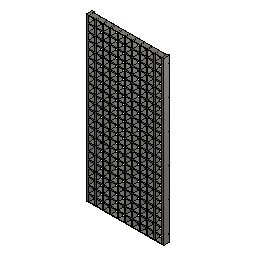
Garlic220 frame (Autodesk Fusion 360 design; units mm, degrees)
Autodesk Fusion 360 part; units mm, degrees
(part 1 of 5)
sketch "Sketch1" plane through (0, 0, 0) normal (0, 0, 1) x (1, 0, 0)
  line L0 (-100, 220) -> (100, 220)
  line L1 (100, 220) -> (100, -220)
  line L2 (100, -220) -> (-100, -220)
  line L3 (-100, -220) -> (-100, 220)
  line L4 (-100, 220) -> (100, -220) construction
  line L5 (100, 220) -> (-100, -220) construction
  line L6 (-100, -220) -> (-80, -220) construction
  line L7 (-80, -220) -> (-80, -200) construction
  line L8 (-80, -200) -> (-100, -200) construction
  line L9 (-100, -200) -> (-100, -220) construction
  line L10 (-98.5, -218.5) -> (-81.5, -218.5)
  line L11 (-81.5, -218.5) -> (-81.5, -201.5)
  line L12 (-81.5, -201.5) -> (-98.5, -201.5)
  line L13 (-98.5, -201.5) -> (-98.5, -218.5)
  line L14 (-61.5, -201.5) -> (-78.5, -201.5)
  line L15 (-61.5, -218.5) -> (-61.5, -201.5)
  line L16 (-78.5, -201.5) -> (-78.5, -218.5)
  line L17 (-78.5, -218.5) -> (-61.5, -218.5)
  line L18 (-60, -220) -> (-60, -200) construction
  line L19 (-60, -200) -> (-80, -200) construction
  line L20 (-41.5, -201.5) -> (-58.5, -201.5)
  line L21 (-41.5, -218.5) -> (-41.5, -201.5)
  line L22 (-58.5, -201.5) -> (-58.5, -218.5)
  line L23 (-58.5, -218.5) -> (-41.5, -218.5)
  line L24 (-40, -220) -> (-40, -200) construction
  line L25 (-40, -200) -> (-60, -200) construction
  line L26 (-21.5, -201.5) -> (-38.5, -201.5)
  line L27 (-21.5, -218.5) -> (-21.5, -201.5)
  line L28 (-38.5, -201.5) -> (-38.5, -218.5)
  line L29 (-38.5, -218.5) -> (-21.5, -218.5)
  line L30 (-20, -220) -> (-20, -200) construction
  line L31 (-20, -200) -> (-40, -200) construction
  line L32 (-1.5, -201.5) -> (-18.5, -201.5)
  line L33 (-1.5, -218.5) -> (-1.5, -201.5)
  line L34 (-18.5, -201.5) -> (-18.5, -218.5)
  line L35 (-18.5, -218.5) -> (-1.5, -218.5)
  line L36 (0, -220) -> (0, -200) construction
  line L37 (0, -200) -> (-20, -200) construction
  line L38 (18.5, -201.5) -> (1.5, -201.5)
  line L39 (18.5, -218.5) -> (18.5, -201.5)
  line L40 (1.5, -201.5) -> (1.5, -218.5)
  line L41 (1.5, -218.5) -> (18.5, -218.5)
  line L42 (20, -220) -> (20, -200) construction
  line L43 (20, -200) -> (0, -200) construction
  line L44 (38.5, -201.5) -> (21.5, -201.5)
  line L45 (38.5, -218.5) -> (38.5, -201.5)
  line L46 (21.5, -201.5) -> (21.5, -218.5)
  line L47 (21.5, -218.5) -> (38.5, -218.5)
  line L48 (40, -220) -> (40, -200) construction
  line L49 (40, -200) -> (20, -200) construction
  line L50 (58.5, -201.5) -> (41.5, -201.5)
  line L51 (58.5, -218.5) -> (58.5, -201.5)
  line L52 (41.5, -201.5) -> (41.5, -218.5)
  line L53 (41.5, -218.5) -> (58.5, -218.5)
  line L54 (60, -220) -> (60, -200) construction
  line L55 (60, -200) -> (40, -200) construction
  line L56 (78.5, -201.5) -> (61.5, -201.5)
  line L57 (78.5, -218.5) -> (78.5, -201.5)
  line L58 (61.5, -201.5) -> (61.5, -218.5)
  line L59 (61.5, -218.5) -> (78.5, -218.5)
  line L60 (80, -220) -> (80, -200) construction
  line L61 (80, -200) -> (60, -200) construction
  line L62 (98.5, -201.5) -> (81.5, -201.5)
  line L63 (98.5, -218.5) -> (98.5, -201.5)
  line L64 (81.5, -201.5) -> (81.5, -218.5)
  line L65 (81.5, -218.5) -> (98.5, -218.5)
  line L66 (100, -220) -> (100, -200) construction
  line L67 (100, -200) -> (80, -200) construction
  line L68 (-81.5, -181.5) -> (-98.5, -181.5)
  line L69 (-81.5, -198.5) -> (-81.5, -181.5)
  line L70 (-98.5, -181.5) -> (-98.5, -198.5)
  line L71 (-98.5, -198.5) -> (-81.5, -198.5)
  line L72 (-80, -200) -> (-80, -180) construction
  line L73 (-80, -180) -> (-100, -180) construction
  line L74 (-61.5, -181.5) -> (-78.5, -181.5)
  line L75 (-61.5, -198.5) -> (-61.5, -181.5)
  line L76 (-78.5, -181.5) -> (-78.5, -198.5)
  line L77 (-78.5, -198.5) -> (-61.5, -198.5)
  line L78 (-60, -200) -> (-60, -180) construction
  line L79 (-60, -180) -> (-80, -180) construction
  line L80 (-41.5, -181.5) -> (-58.5, -181.5)
  line L81 (-41.5, -198.5) -> (-41.5, -181.5)
  line L82 (-58.5, -181.5) -> (-58.5, -198.5)
  line L83 (-58.5, -198.5) -> (-41.5, -198.5)
  line L84 (-40, -200) -> (-40, -180) construction
  line L85 (-40, -180) -> (-60, -180) construction
  line L86 (-21.5, -181.5) -> (-38.5, -181.5)
  line L87 (-21.5, -198.5) -> (-21.5, -181.5)
  line L88 (-38.5, -181.5) -> (-38.5, -198.5)
  line L89 (-38.5, -198.5) -> (-21.5, -198.5)
  line L90 (-20, -200) -> (-20, -180) construction
  line L91 (-20, -180) -> (-40, -180) construction
  line L92 (-1.5, -181.5) -> (-18.5, -181.5)
  line L93 (-1.5, -198.5) -> (-1.5, -181.5)
  line L94 (-18.5, -181.5) -> (-18.5, -198.5)
  line L95 (-18.5, -198.5) -> (-1.5, -198.5)
  line L96 (0, -200) -> (0, -180) construction
  line L97 (0, -180) -> (-20, -180) construction
  line L98 (18.5, -181.5) -> (1.5, -181.5)
  line L99 (18.5, -198.5) -> (18.5, -181.5)
  line L100 (1.5, -181.5) -> (1.5, -198.5)
  line L101 (1.5, -198.5) -> (18.5, -198.5)
  line L102 (20, -200) -> (20, -180) construction
  line L103 (20, -180) -> (0, -180) construction
  line L104 (38.5, -181.5) -> (21.5, -181.5)
  line L105 (38.5, -198.5) -> (38.5, -181.5)
  line L106 (21.5, -181.5) -> (21.5, -198.5)
  line L107 (21.5, -198.5) -> (38.5, -198.5)
  line L108 (40, -200) -> (40, -180) construction
  line L109 (40, -180) -> (20, -180) construction
  line L110 (58.5, -181.5) -> (41.5, -181.5)
  line L111 (58.5, -198.5) -> (58.5, -181.5)
  line L112 (41.5, -181.5) -> (41.5, -198.5)
  line L113 (41.5, -198.5) -> (58.5, -198.5)
  line L114 (60, -200) -> (60, -180) construction
  line L115 (60, -180) -> (40, -180) construction
  line L116 (78.5, -181.5) -> (61.5, -181.5)
  line L117 (78.5, -198.5) -> (78.5, -181.5)
  line L118 (61.5, -181.5) -> (61.5, -198.5)
  line L119 (61.5, -198.5) -> (78.5, -198.5)
  line L120 (80, -200) -> (80, -180) construction
  line L121 (80, -180) -> (60, -180) construction
  line L122 (98.5, -181.5) -> (81.5, -181.5)
  line L123 (98.5, -198.5) -> (98.5, -181.5)
  line L124 (81.5, -181.5) -> (81.5, -198.5)
  line L125 (81.5, -198.5) -> (98.5, -198.5)
  line L126 (100, -200) -> (100, -180) construction
  line L127 (100, -180) -> (80, -180) construction
  line L128 (-81.5, -161.5) -> (-98.5, -161.5)
  line L129 (-81.5, -178.5) -> (-81.5, -161.5)
  line L130 (-98.5, -161.5) -> (-98.5, -178.5)
  line L131 (-98.5, -178.5) -> (-81.5, -178.5)
  line L132 (-80, -180) -> (-80, -160) construction
  line L133 (-80, -160) -> (-100, -160) construction
  line L134 (-61.5, -161.5) -> (-78.5, -161.5)
  line L135 (-61.5, -178.5) -> (-61.5, -161.5)
  line L136 (-78.5, -161.5) -> (-78.5, -178.5)
  line L137 (-78.5, -178.5) -> (-61.5, -178.5)
  line L138 (-60, -180) -> (-60, -160) construction
  line L139 (-60, -160) -> (-80, -160) construction
  line L140 (-41.5, -161.5) -> (-58.5, -161.5)
  line L141 (-41.5, -178.5) -> (-41.5, -161.5)
  line L142 (-58.5, -161.5) -> (-58.5, -178.5)
  line L143 (-58.5, -178.5) -> (-41.5, -178.5)
  line L144 (-40, -180) -> (-40, -160) construction
  line L145 (-40, -160) -> (-60, -160) construction
  line L146 (-21.5, -161.5) -> (-38.5, -161.5)
  line L147 (-21.5, -178.5) -> (-21.5, -161.5)
  line L148 (-38.5, -161.5) -> (-38.5, -178.5)
  line L149 (-38.5, -178.5) -> (-21.5, -178.5)
  line L150 (-20, -180) -> (-20, -160) construction
  line L151 (-20, -160) -> (-40, -160) construction
  line L152 (-1.5, -161.5) -> (-18.5, -161.5)
  line L153 (-1.5, -178.5) -> (-1.5, -161.5)
  line L154 (-18.5, -161.5) -> (-18.5, -178.5)
  line L155 (-18.5, -178.5) -> (-1.5, -178.5)
  line L156 (0, -180) -> (0, -160) construction
  line L157 (0, -160) -> (-20, -160) construction
  line L158 (18.5, -161.5) -> (1.5, -161.5)
  line L159 (18.5, -178.5) -> (18.5, -161.5)
  line L160 (1.5, -161.5) -> (1.5, -178.5)
  line L161 (1.5, -178.5) -> (18.5, -178.5)
  line L162 (20, -180) -> (20, -160) construction
  line L163 (20, -160) -> (0, -160) construction
  line L164 (38.5, -161.5) -> (21.5, -161.5)
  line L165 (38.5, -178.5) -> (38.5, -161.5)
  line L166 (21.5, -161.5) -> (21.5, -178.5)
  line L167 (21.5, -178.5) -> (38.5, -178.5)
  line L168 (40, -180) -> (40, -160) construction
  line L169 (40, -160) -> (20, -160) construction
  line L170 (58.5, -161.5) -> (41.5, -161.5)
  line L171 (58.5, -178.5) -> (58.5, -161.5)
  line L172 (41.5, -161.5) -> (41.5, -178.5)
  line L173 (41.5, -178.5) -> (58.5, -178.5)
  line L174 (60, -180) -> (60, -160) construction
  line L175 (60, -160) -> (40, -160) construction
  line L176 (78.5, -161.5) -> (61.5, -161.5)
  line L177 (78.5, -178.5) -> (78.5, -161.5)
  line L178 (61.5, -161.5) -> (61.5, -178.5)
  line L179 (61.5, -178.5) -> (78.5, -178.5)
  line L180 (80, -180) -> (80, -160) construction
  line L181 (80, -160) -> (60, -160) construction
  line L182 (98.5, -161.5) -> (81.5, -161.5)
  line L183 (98.5, -178.5) -> (98.5, -161.5)
  line L184 (81.5, -161.5) -> (81.5, -178.5)
  line L185 (81.5, -178.5) -> (98.5, -178.5)
  line L186 (100, -180) -> (100, -160) construction
  line L187 (100, -160) -> (80, -160) construction
  line L188 (-81.5, -141.5) -> (-98.5, -141.5)
  line L189 (-81.5, -158.5) -> (-81.5, -141.5)
  line L190 (-98.5, -141.5) -> (-98.5, -158.5)
  line L191 (-98.5, -158.5) -> (-81.5, -158.5)
  line L192 (-80, -160) -> (-80, -140) construction
  line L193 (-80, -140) -> (-100, -140) construction
  line L194 (-61.5, -141.5) -> (-78.5, -141.5)
  line L195 (-61.5, -158.5) -> (-61.5, -141.5)
  line L196 (-78.5, -141.5) -> (-78.5, -158.5)
  line L197 (-78.5, -158.5) -> (-61.5, -158.5)
  line L198 (-60, -160) -> (-60, -140) construction
  line L199 (-60, -140) -> (-80, -140) construction
  line L200 (-41.5, -141.5) -> (-58.5, -141.5)
  line L201 (-41.5, -158.5) -> (-41.5, -141.5)
  line L202 (-58.5, -141.5) -> (-58.5, -158.5)
  line L203 (-58.5, -158.5) -> (-41.5, -158.5)
  line L204 (-40, -160) -> (-40, -140) construction
  line L205 (-40, -140) -> (-60, -140) construction
  line L206 (-21.5, -141.5) -> (-38.5, -141.5)
  line L207 (-21.5, -158.5) -> (-21.5, -141.5)
  line L208 (-38.5, -141.5) -> (-38.5, -158.5)
  line L209 (-38.5, -158.5) -> (-21.5, -158.5)
  line L210 (-20, -160) -> (-20, -140) construction
  line L211 (-20, -140) -> (-40, -140) construction
  line L212 (-1.5, -141.5) -> (-18.5, -141.5)
  line L213 (-1.5, -158.5) -> (-1.5, -141.5)
  line L214 (-18.5, -141.5) -> (-18.5, -158.5)
  line L215 (-18.5, -158.5) -> (-1.5, -158.5)
  line L216 (0, -160) -> (0, -140) construction
  line L217 (0, -140) -> (-20, -140) construction
  line L218 (18.5, -141.5) -> (1.5, -141.5)
  line L219 (18.5, -158.5) -> (18.5, -141.5)
  line L220 (1.5, -141.5) -> (1.5, -158.5)
  line L221 (1.5, -158.5) -> (18.5, -158.5)
  line L222 (20, -160) -> (20, -140) construction
  line L223 (20, -140) -> (0, -140) construction
  line L224 (38.5, -141.5) -> (21.5, -141.5)
  line L225 (38.5, -158.5) -> (38.5, -141.5)
  line L226 (21.5, -141.5) -> (21.5, -158.5)
  line L227 (21.5, -158.5) -> (38.5, -158.5)
  line L228 (40, -160) -> (40, -140) construction
  line L229 (40, -140) -> (20, -140) construction
  line L230 (58.5, -141.5) -> (41.5, -141.5)
  line L231 (58.5, -158.5) -> (58.5, -141.5)
  line L232 (41.5, -141.5) -> (41.5, -158.5)
  line L233 (41.5, -158.5) -> (58.5, -158.5)
  line L234 (60, -160) -> (60, -140) construction
  line L235 (60, -140) -> (40, -140) construction
  line L236 (78.5, -141.5) -> (61.5, -141.5)
  line L237 (78.5, -158.5) -> (78.5, -141.5)
  line L238 (61.5, -141.5) -> (61.5, -158.5)
  line L239 (61.5, -158.5) -> (78.5, -158.5)
  line L240 (80, -160) -> (80, -140) construction
  line L241 (80, -140) -> (60, -140) construction
  line L242 (98.5, -141.5) -> (81.5, -141.5)
  line L243 (98.5, -158.5) -> (98.5, -141.5)
  line L244 (81.5, -141.5) -> (81.5, -158.5)
  line L245 (81.5, -158.5) -> (98.5, -158.5)
  line L246 (100, -160) -> (100, -140) construction
  line L247 (100, -140) -> (80, -140) construction
  line L248 (-81.5, -121.5) -> (-98.5, -121.5)
  line L249 (-81.5, -138.5) -> (-81.5, -121.5)
  line L250 (-98.5, -121.5) -> (-98.5, -138.5)
  line L251 (-98.5, -138.5) -> (-81.5, -138.5)
  line L252 (-80, -140) -> (-80, -120) construction
  line L253 (-80, -120) -> (-100, -120) construction
  line L254 (-61.5, -121.5) -> (-78.5, -121.5)
  line L255 (-61.5, -138.5) -> (-61.5, -121.5)
  line L256 (-78.5, -121.5) -> (-78.5, -138.5)
  line L257 (-78.5, -138.5) -> (-61.5, -138.5)
  line L258 (-60, -140) -> (-60, -120) construction
  line L259 (-60, -120) -> (-80, -120) construction
  line L260 (-41.5, -121.5) -> (-58.5, -121.5)
  line L261 (-41.5, -138.5) -> (-41.5, -121.5)
  line L262 (-58.5, -121.5) -> (-58.5, -138.5)
  line L263 (-58.5, -138.5) -> (-41.5, -138.5)
  line L264 (-40, -140) -> (-40, -120) construction
  line L265 (-40, -120) -> (-60, -120) construction
  line L266 (-21.5, -121.5) -> (-38.5, -121.5)
  line L267 (-21.5, -138.5) -> (-21.5, -121.5)
  line L268 (-38.5, -121.5) -> (-38.5, -138.5)
  line L269 (-38.5, -138.5) -> (-21.5, -138.5)
  line L270 (-20, -140) -> (-20, -120) construction
  line L271 (-20, -120) -> (-40, -120) construction
  line L272 (-1.5, -121.5) -> (-18.5, -121.5)
  line L273 (-1.5, -138.5) -> (-1.5, -121.5)
  line L274 (-18.5, -121.5) -> (-18.5, -138.5)
  line L275 (-18.5, -138.5) -> (-1.5, -138.5)
  line L276 (0, -140) -> (0, -120) construction
  line L277 (0, -120) -> (-20, -120) construction
  line L278 (18.5, -121.5) -> (1.5, -121.5)
  line L279 (18.5, -138.5) -> (18.5, -121.5)
  line L280 (1.5, -121.5) -> (1.5, -138.5)
  line L281 (1.5, -138.5) -> (18.5, -138.5)
  line L282 (20, -140) -> (20, -120) construction
  line L283 (20, -120) -> (0, -120) construction
  line L284 (38.5, -121.5) -> (21.5, -121.5)
  line L285 (38.5, -138.5) -> (38.5, -121.5)
  line L286 (21.5, -121.5) -> (21.5, -138.5)
  line L287 (21.5, -138.5) -> (38.5, -138.5)
  line L288 (40, -140) -> (40, -120) construction
  line L289 (40, -120) -> (20, -120) construction
  line L290 (58.5, -121.5) -> (41.5, -121.5)
  line L291 (58.5, -138.5) -> (58.5, -121.5)
  line L292 (41.5, -121.5) -> (41.5, -138.5)
  line L293 (41.5, -138.5) -> (58.5, -138.5)
  line L294 (60, -140) -> (60, -120) construction
  line L295 (60, -120) -> (40, -120) construction
  line L296 (78.5, -121.5) -> (61.5, -121.5)
  line L297 (78.5, -138.5) -> (78.5, -121.5)
  line L298 (61.5, -121.5) -> (61.5, -138.5)
  line L299 (61.5, -138.5) -> (78.5, -138.5)
  line L300 (80, -140) -> (80, -120) construction
  line L301 (80, -120) -> (60, -120) construction
  line L302 (98.5, -121.5) -> (81.5, -121.5)
  line L303 (98.5, -138.5) -> (98.5, -121.5)
  line L304 (81.5, -121.5) -> (81.5, -138.5)
  line L305 (81.5, -138.5) -> (98.5, -138.5)
  line L306 (100, -140) -> (100, -120) construction
  line L307 (100, -120) -> (80, -120) construction
  line L308 (-81.5, -101.5) -> (-98.5, -101.5)
  line L309 (-81.5, -118.5) -> (-81.5, -101.5)
  line L310 (-98.5, -101.5) -> (-98.5, -118.5)
  line L311 (-98.5, -118.5) -> (-81.5, -118.5)
  line L312 (-80, -120) -> (-80, -100) construction
  line L313 (-80, -100) -> (-100, -100) construction
  line L314 (-61.5, -101.5) -> (-78.5, -101.5)
  line L315 (-61.5, -118.5) -> (-61.5, -101.5)
  line L316 (-78.5, -101.5) -> (-78.5, -118.5)
  line L317 (-78.5, -118.5) -> (-61.5, -118.5)
  line L318 (-60, -120) -> (-60, -100) construction
  line L319 (-60, -100) -> (-80, -100) construction
  line L320 (-41.5, -101.5) -> (-58.5, -101.5)
  line L321 (-41.5, -118.5) -> (-41.5, -101.5)
  line L322 (-58.5, -101.5) -> (-58.5, -118.5)
  line L323 (-58.5, -118.5) -> (-41.5, -118.5)
  line L324 (-40, -120) -> (-40, -100) construction
  line L325 (-40, -100) -> (-60, -100) construction
  line L326 (-21.5, -101.5) -> (-38.5, -101.5)
  line L327 (-21.5, -118.5) -> (-21.5, -101.5)
  line L328 (-38.5, -101.5) -> (-38.5, -118.5)
  line L329 (-38.5, -118.5) -> (-21.5, -118.5)
  line L330 (-20, -120) -> (-20, -100) construction
  line L331 (-20, -100) -> (-40, -100) construction
  line L332 (-1.5, -101.5) -> (-18.5, -101.5)
  line L333 (-1.5, -118.5) -> (-1.5, -101.5)
  line L334 (-18.5, -101.5) -> (-18.5, -118.5)
  line L335 (-18.5, -118.5) -> (-1.5, -118.5)
  line L336 (0, -120) -> (0, -100) construction
  line L337 (0, -100) -> (-20, -100) construction
  line L338 (18.5, -101.5) -> (1.5, -101.5)
  line L339 (18.5, -118.5) -> (18.5, -101.5)
  line L340 (1.5, -101.5) -> (1.5, -118.5)
  line L341 (1.5, -118.5) -> (18.5, -118.5)
  line L342 (20, -120) -> (20, -100) construction
  line L343 (20, -100) -> (0, -100) construction
  line L344 (38.5, -101.5) -> (21.5, -101.5)
  line L345 (38.5, -118.5) -> (38.5, -101.5)
  line L346 (21.5, -101.5) -> (21.5, -118.5)
  line L347 (21.5, -118.5) -> (38.5, -118.5)
  line L348 (40, -120) -> (40, -100) construction
  line L349 (40, -100) -> (20, -100) construction
  line L350 (58.5, -101.5) -> (41.5, -101.5)
  line L351 (58.5, -118.5) -> (58.5, -101.5)
  line L352 (41.5, -101.5) -> (41.5, -118.5)
  line L353 (41.5, -118.5) -> (58.5, -118.5)
  line L354 (60, -120) -> (60, -100) construction
  line L355 (60, -100) -> (40, -100) construction
  line L356 (78.5, -101.5) -> (61.5, -101.5)
  line L357 (78.5, -118.5) -> (78.5, -101.5)
  line L358 (61.5, -101.5) -> (61.5, -118.5)
  line L359 (61.5, -118.5) -> (78.5, -118.5)
  line L360 (80, -120) -> (80, -100) construction
  line L361 (80, -100) -> (60, -100) construction
  line L362 (98.5, -101.5) -> (81.5, -101.5)
  line L363 (98.5, -118.5) -> (98.5, -101.5)
  line L364 (81.5, -101.5) -> (81.5, -118.5)
  line L365 (81.5, -118.5) -> (98.5, -118.5)
  line L366 (100, -120) -> (100, -100) construction
  line L367 (100, -100) -> (80, -100) construction
  line L368 (-81.5, -81.5) -> (-98.5, -81.5)
  line L369 (-81.5, -98.5) -> (-81.5, -81.5)
  line L370 (-98.5, -81.5) -> (-98.5, -98.5)
  line L371 (-98.5, -98.5) -> (-81.5, -98.5)
  line L372 (-80, -100) -> (-80, -80) construction
  line L373 (-80, -80) -> (-100, -80) construction
  line L374 (-61.5, -81.5) -> (-78.5, -81.5)
  line L375 (-61.5, -98.5) -> (-61.5, -81.5)
  line L376 (-78.5, -81.5) -> (-78.5, -98.5)
  line L377 (-78.5, -98.5) -> (-61.5, -98.5)
  line L378 (-60, -100) -> (-60, -80) construction
  line L379 (-60, -80) -> (-80, -80) construction
  line L380 (-41.5, -81.5) -> (-58.5, -81.5)
  line L381 (-41.5, -98.5) -> (-41.5, -81.5)
  line L382 (-58.5, -81.5) -> (-58.5, -98.5)
  line L383 (-58.5, -98.5) -> (-41.5, -98.5)
  line L384 (-40, -100) -> (-40, -80) construction
  line L385 (-40, -80) -> (-60, -80) construction
  line L386 (-21.5, -81.5) -> (-38.5, -81.5)
  line L387 (-21.5, -98.5) -> (-21.5, -81.5)
  line L388 (-38.5, -81.5) -> (-38.5, -98.5)
  line L389 (-38.5, -98.5) -> (-21.5, -98.5)
  line L390 (-20, -100) -> (-20, -80) construction
  line L391 (-20, -80) -> (-40, -80) construction
  line L392 (-1.5, -81.5) -> (-18.5, -81.5)
  line L393 (-1.5, -98.5) -> (-1.5, -81.5)
  line L394 (-18.5, -81.5) -> (-18.5, -98.5)
  line L395 (-18.5, -98.5) -> (-1.5, -98.5)
  line L396 (0, -100) -> (0, -80) construction
  line L397 (0, -80) -> (-20, -80) construction
  line L398 (18.5, -81.5) -> (1.5, -81.5)
  line L399 (18.5, -98.5) -> (18.5, -81.5)
  line L400 (1.5, -81.5) -> (1.5, -98.5)
  line L401 (1.5, -98.5) -> (18.5, -98.5)
  line L402 (20, -100) -> (20, -80) construction
  line L403 (20, -80) -> (0, -80) construction
  line L404 (38.5, -81.5) -> (21.5, -81.5)
  line L405 (38.5, -98.5) -> (38.5, -81.5)
  line L406 (21.5, -81.5) -> (21.5, -98.5)
  line L407 (21.5, -98.5) -> (38.5, -98.5)
  line L408 (40, -100) -> (40, -80) construction
  line L409 (40, -80) -> (20, -80) construction
  line L410 (58.5, -81.5) -> (41.5, -81.5)
  line L411 (58.5, -98.5) -> (58.5, -81.5)
  line L412 (41.5, -81.5) -> (41.5, -98.5)
  line L413 (41.5, -98.5) -> (58.5, -98.5)
  line L414 (60, -100) -> (60, -80) construction
  line L415 (60, -80) -> (40, -80) construction
  line L416 (78.5, -81.5) -> (61.5, -81.5)
  line L417 (78.5, -98.5) -> (78.5, -81.5)
  line L418 (61.5, -81.5) -> (61.5, -98.5)
  line L419 (61.5, -98.5) -> (78.5, -98.5)
  line L420 (80, -100) -> (80, -80) construction
  line L421 (80, -80) -> (60, -80) construction
  line L422 (98.5, -81.5) -> (81.5, -81.5)
  line L423 (98.5, -98.5) -> (98.5, -81.5)
  line L424 (81.5, -81.5) -> (81.5, -98.5)
  line L425 (81.5, -98.5) -> (98.5, -98.5)
  line L426 (100, -100) -> (100, -80) construction
  line L427 (100, -80) -> (80, -80) construction
  line L428 (-81.5, -61.5) -> (-98.5, -61.5)
  line L429 (-81.5, -78.5) -> (-81.5, -61.5)
  line L430 (-98.5, -61.5) -> (-98.5, -78.5)
  line L431 (-98.5, -78.5) -> (-81.5, -78.5)
  line L432 (-80, -80) -> (-80, -60) construction
  line L433 (-80, -60) -> (-100, -60) construction
  line L434 (-61.5, -61.5) -> (-78.5, -61.5)
  line L435 (-61.5, -78.5) -> (-61.5, -61.5)
  line L436 (-78.5, -61.5) -> (-78.5, -78.5)
  line L437 (-78.5, -78.5) -> (-61.5, -78.5)
  line L438 (-60, -80) -> (-60, -60) construction
  line L439 (-60, -60) -> (-80, -60) construction
  line L440 (-41.5, -61.5) -> (-58.5, -61.5)
  line L441 (-41.5, -78.5) -> (-41.5, -61.5)
  line L442 (-58.5, -61.5) -> (-58.5, -78.5)
  line L443 (-58.5, -78.5) -> (-41.5, -78.5)
  line L444 (-40, -80) -> (-40, -60) construction
  line L445 (-40, -60) -> (-60, -60) construction
  line L446 (-21.5, -61.5) -> (-38.5, -61.5)
  line L447 (-21.5, -78.5) -> (-21.5, -61.5)
  line L448 (-38.5, -61.5) -> (-38.5, -78.5)
  line L449 (-38.5, -78.5) -> (-21.5, -78.5)
  line L450 (-20, -80) -> (-20, -60) construction
  line L451 (-20, -60) -> (-40, -60) construction
  line L452 (-1.5, -61.5) -> (-18.5, -61.5)
  line L453 (-1.5, -78.5) -> (-1.5, -61.5)
  line L454 (-18.5, -61.5) -> (-18.5, -78.5)
  line L455 (-18.5, -78.5) -> (-1.5, -78.5)
  line L456 (0, -80) -> (0, -60) construction
  line L457 (0, -60) -> (-20, -60) construction
  line L458 (18.5, -61.5) -> (1.5, -61.5)
  line L459 (18.5, -78.5) -> (18.5, -61.5)
  line L460 (1.5, -61.5) -> (1.5, -78.5)
  line L461 (1.5, -78.5) -> (18.5, -78.5)
  line L462 (20, -80) -> (20, -60) construction
  line L463 (20, -60) -> (0, -60) construction
  line L464 (38.5, -61.5) -> (21.5, -61.5)
  line L465 (38.5, -78.5) -> (38.5, -61.5)
  line L466 (21.5, -61.5) -> (21.5, -78.5)
  line L467 (21.5, -78.5) -> (38.5, -78.5)
  line L468 (40, -80) -> (40, -60) construction
  line L469 (40, -60) -> (20, -60) construction
  line L470 (58.5, -61.5) -> (41.5, -61.5)
  line L471 (58.5, -78.5) -> (58.5, -61.5)
  line L472 (41.5, -61.5) -> (41.5, -78.5)
  line L473 (41.5, -78.5) -> (58.5, -78.5)
  line L474 (60, -80) -> (60, -60) construction
  line L475 (60, -60) -> (40, -60) construction
  line L476 (78.5, -61.5) -> (61.5, -61.5)
  line L477 (78.5, -78.5) -> (78.5, -61.5)
  line L478 (61.5, -61.5) -> (61.5, -78.5)
  line L479 (61.5, -78.5) -> (78.5, -78.5)
  line L480 (80, -80) -> (80, -60) construction
  line L481 (80, -60) -> (60, -60) construction
  line L482 (98.5, -61.5) -> (81.5, -61.5)
  line L483 (98.5, -78.5) -> (98.5, -61.5)
  line L484 (81.5, -61.5) -> (81.5, -78.5)
  line L485 (81.5, -78.5) -> (98.5, -78.5)
  line L486 (100, -80) -> (100, -60) construction
  line L487 (100, -60) -> (80, -60) construction
  line L488 (-81.5, -41.5) -> (-98.5, -41.5)
  line L489 (-81.5, -58.5) -> (-81.5, -41.5)
  line L490 (-98.5, -41.5) -> (-98.5, -58.5)
  line L491 (-98.5, -58.5) -> (-81.5, -58.5)
  line L492 (-80, -60) -> (-80, -40) construction
  line L493 (-80, -40) -> (-100, -40) construction
  line L494 (-61.5, -41.5) -> (-78.5, -41.5)
  line L495 (-61.5, -58.5) -> (-61.5, -41.5)
  line L496 (-78.5, -41.5) -> (-78.5, -58.5)
  line L497 (-78.5, -58.5) -> (-61.5, -58.5)
  line L498 (-60, -60) -> (-60, -40) construction
  line L499 (-60, -40) -> (-80, -40) construction
  line L500 (-41.5, -41.5) -> (-58.5, -41.5)
  line L501 (-41.5, -58.5) -> (-41.5, -41.5)
  line L502 (-58.5, -41.5) -> (-58.5, -58.5)
  line L503 (-58.5, -58.5) -> (-41.5, -58.5)
  line L504 (-40, -60) -> (-40, -40) construction
  line L505 (-40, -40) -> (-60, -40) construction
  line L506 (-21.5, -41.5) -> (-38.5, -41.5)
  line L507 (-21.5, -58.5) -> (-21.5, -41.5)
  line L508 (-38.5, -41.5) -> (-38.5, -58.5)
  line L509 (-38.5, -58.5) -> (-21.5, -58.5)
  line L510 (-20, -60) -> (-20, -40) construction
  line L511 (-20, -40) -> (-40, -40) construction
  line L512 (-1.5, -41.5) -> (-18.5, -41.5)
  line L513 (-1.5, -58.5) -> (-1.5, -41.5)
  line L514 (-18.5, -41.5) -> (-18.5, -58.5)
  line L515 (-18.5, -58.5) -> (-1.5, -58.5)
  line L516 (0, -60) -> (0, -40) construction
  line L517 (0, -40) -> (-20, -40) construction
  line L518 (18.5, -41.5) -> (1.5, -41.5)
  line L519 (18.5, -58.5) -> (18.5, -41.5)
  line L520 (1.5, -41.5) -> (1.5, -58.5)
  line L521 (1.5, -58.5) -> (18.5, -58.5)
  line L522 (20, -60) -> (20, -40) construction
  line L523 (20, -40) -> (0, -40) construction
  line L524 (38.5, -41.5) -> (21.5, -41.5)
  line L525 (38.5, -58.5) -> (38.5, -41.5)
  line L526 (21.5, -41.5) -> (21.5, -58.5)
  line L527 (21.5, -58.5) -> (38.5, -58.5)
  line L528 (40, -60) -> (40, -40) construction
  line L529 (40, -40) -> (20, -40) construction
  line L530 (58.5, -41.5) -> (41.5, -41.5)
  line L531 (58.5, -58.5) -> (58.5, -41.5)
  line L532 (41.5, -41.5) -> (41.5, -58.5)
  line L533 (41.5, -58.5) -> (58.5, -58.5)
  line L534 (60, -60) -> (60, -40) construction
  line L535 (60, -40) -> (40, -40) construction
  line L536 (78.5, -41.5) -> (61.5, -41.5)
  line L537 (78.5, -58.5) -> (78.5, -41.5)
  line L538 (61.5, -41.5) -> (61.5, -58.5)
  line L539 (61.5, -58.5) -> (78.5, -58.5)
  line L540 (80, -60) -> (80, -40) construction
  line L541 (80, -40) -> (60, -40) construction
  line L542 (98.5, -41.5) -> (81.5, -41.5)
  line L543 (98.5, -58.5) -> (98.5, -41.5)
  line L544 (81.5, -41.5) -> (81.5, -58.5)
  line L545 (81.5, -58.5) -> (98.5, -58.5)
  line L546 (100, -60) -> (100, -40) construction
  line L547 (100, -40) -> (80, -40) construction
  line L548 (-81.5, -21.5) -> (-98.5, -21.5)
  line L549 (-81.5, -38.5) -> (-81.5, -21.5)
  line L550 (-98.5, -21.5) -> (-98.5, -38.5)
  line L551 (-98.5, -38.5) -> (-81.5, -38.5)
  line L552 (-80, -40) -> (-80, -20) construction
  line L553 (-80, -20) -> (-100, -20) construction
  line L554 (-61.5, -21.5) -> (-78.5, -21.5)
  line L555 (-61.5, -38.5) -> (-61.5, -21.5)
  line L556 (-78.5, -21.5) -> (-78.5, -38.5)
  line L557 (-78.5, -38.5) -> (-61.5, -38.5)
  line L558 (-60, -40) -> (-60, -20) construction
  line L559 (-60, -20) -> (-80, -20) construction
  line L560 (-41.5, -21.5) -> (-58.5, -21.5)
  line L561 (-41.5, -38.5) -> (-41.5, -21.5)
  line L562 (-58.5, -21.5) -> (-58.5, -38.5)
  line L563 (-58.5, -38.5) -> (-41.5, -38.5)
  line L564 (-40, -40) -> (-40, -20) construction
  line L565 (-40, -20) -> (-60, -20) construction
  line L566 (-21.5, -21.5) -> (-38.5, -21.5)
  line L567 (-21.5, -38.5) -> (-21.5, -21.5)
  line L568 (-38.5, -21.5) -> (-38.5, -38.5)
  line L569 (-38.5, -38.5) -> (-21.5, -38.5)
  line L570 (-20, -40) -> (-20, -20) construction
  line L571 (-20, -20) -> (-40, -20) construction
  line L572 (-1.5, -21.5) -> (-18.5, -21.5)
  line L573 (-1.5, -38.5) -> (-1.5, -21.5)
  line L574 (-18.5, -21.5) -> (-18.5, -38.5)
  line L575 (-18.5, -38.5) -> (-1.5, -38.5)
  line L576 (0, -40) -> (0, -20) construction
  line L577 (0, -20) -> (-20, -20) construction
  line L578 (18.5, -21.5) -> (1.5, -21.5)
  line L579 (18.5, -38.5) -> (18.5, -21.5)
  line L580 (1.5, -21.5) -> (1.5, -38.5)
  line L581 (1.5, -38.5) -> (18.5, -38.5)
  line L582 (20, -40) -> (20, -20) construction
  line L583 (20, -20) -> (0, -20) construction
  line L584 (38.5, -21.5) -> (21.5, -21.5)
  line L585 (38.5, -38.5) -> (38.5, -21.5)
  line L586 (21.5, -21.5) -> (21.5, -38.5)
  line L587 (21.5, -38.5) -> (38.5, -38.5)
  line L588 (40, -40) -> (40, -20) construction
  line L589 (40, -20) -> (20, -20) construction
  line L590 (58.5, -21.5) -> (41.5, -21.5)
  line L591 (58.5, -38.5) -> (58.5, -21.5)
  line L592 (41.5, -21.5) -> (41.5, -38.5)
  line L593 (41.5, -38.5) -> (58.5, -38.5)
  line L594 (60, -40) -> (60, -20) construction
  line L595 (60, -20) -> (40, -20) construction
  line L596 (78.5, -21.5) -> (61.5, -21.5)
  line L597 (78.5, -38.5) -> (78.5, -21.5)
  line L598 (61.5, -21.5) -> (61.5, -38.5)
  line L599 (61.5, -38.5) -> (78.5, -38.5)
  line L600 (80, -40) -> (80, -20) construction
  line L601 (80, -20) -> (60, -20) construction
  line L602 (98.5, -21.5) -> (81.5, -21.5)
  line L603 (98.5, -38.5) -> (98.5, -21.5)
  line L604 (81.5, -21.5) -> (81.5, -38.5)
  line L605 (81.5, -38.5) -> (98.5, -38.5)
  line L606 (100, -40) -> (100, -20) construction
  line L607 (100, -20) -> (80, -20) construction
  line L608 (-81.5, -1.5) -> (-98.5, -1.5)
  line L609 (-81.5, -18.5) -> (-81.5, -1.5)
  line L610 (-98.5, -1.5) -> (-98.5, -18.5)
  line L611 (-98.5, -18.5) -> (-81.5, -18.5)
  line L612 (-80, -20) -> (-80, 0) construction
  line L613 (-80, 0) -> (-100, 0) construction
  line L614 (-61.5, -1.5) -> (-78.5, -1.5)
  line L615 (-61.5, -18.5) -> (-61.5, -1.5)
  line L616 (-78.5, -1.5) -> (-78.5, -18.5)
  line L617 (-78.5, -18.5) -> (-61.5, -18.5)
  line L618 (-60, -20) -> (-60, 0) construction
  line L619 (-60, 0) -> (-80, 0) construction
  line L620 (-41.5, -1.5) -> (-58.5, -1.5)
  line L621 (-41.5, -18.5) -> (-41.5, -1.5)
  line L622 (-58.5, -1.5) -> (-58.5, -18.5)
  line L623 (-58.5, -18.5) -> (-41.5, -18.5)
  line L624 (-40, -20) -> (-40, 0) construction
  line L625 (-40, 0) -> (-60, 0) construction
  line L626 (-21.5, -1.5) -> (-38.5, -1.5)
  line L627 (-21.5, -18.5) -> (-21.5, -1.5)
  line L628 (-38.5, -1.5) -> (-38.5, -18.5)
  line L629 (-38.5, -18.5) -> (-21.5, -18.5)
  line L630 (-20, -20) -> (-20, 0) construction
  line L631 (-20, 0) -> (-40, 0) construction
  line L632 (-1.5, -1.5) -> (-18.5, -1.5)
  line L633 (-1.5, -18.5) -> (-1.5, -1.5)
  line L634 (-18.5, -1.5) -> (-18.5, -18.5)
  line L635 (-18.5, -18.5) -> (-1.5, -18.5)
  line L636 (0, -20) -> (0, 0) construction
  line L637 (0, 0) -> (-20, 0) construction
  line L638 (18.5, -1.5) -> (1.5, -1.5)
  line L639 (18.5, -18.5) -> (18.5, -1.5)
  line L640 (1.5, -1.5) -> (1.5, -18.5)
  line L641 (1.5, -18.5) -> (18.5, -18.5)
  line L642 (20, -20) -> (20, 0) construction
  line L643 (20, 0) -> (0, 0) construction
  line L644 (38.5, -1.5) -> (21.5, -1.5)
  line L645 (38.5, -18.5) -> (38.5, -1.5)
  line L646 (21.5, -1.5) -> (21.5, -18.5)
  line L647 (21.5, -18.5) -> (38.5, -18.5)
  line L648 (40, -20) -> (40, 0) construction
  line L649 (40, 0) -> (20, 0) construction
  line L650 (58.5, -1.5) -> (41.5, -1.5)
  line L651 (58.5, -18.5) -> (58.5, -1.5)
  line L652 (41.5, -1.5) -> (41.5, -18.5)
  line L653 (41.5, -18.5) -> (58.5, -18.5)
  line L654 (60, -20) -> (60, 0) construction
  line L655 (60, 0) -> (40, 0) construction
  line L656 (78.5, -1.5) -> (61.5, -1.5)
  line L657 (78.5, -18.5) -> (78.5, -1.5)
  line L658 (61.5, -1.5) -> (61.5, -18.5)
  line L659 (61.5, -18.5) -> (78.5, -18.5)
  line L660 (80, -20) -> (80, 0) construction
  line L661 (80, 0) -> (60, 0) construction
  line L662 (98.5, -1.5) -> (81.5, -1.5)
  line L663 (98.5, -18.5) -> (98.5, -1.5)
  line L664 (81.5, -1.5) -> (81.5, -18.5)
  line L665 (81.5, -18.5) -> (98.5, -18.5)
  line L666 (100, -20) -> (100, 0) construction
  line L667 (100, 0) -> (80, 0) construction
  line L668 (-81.5, 18.5) -> (-98.5, 18.5)
  line L669 (-81.5, 1.5) -> (-81.5, 18.5)
  line L670 (-98.5, 18.5) -> (-98.5, 1.5)
  line L671 (-98.5, 1.5) -> (-81.5, 1.5)
  line L672 (-80, 0) -> (-80, 20) construction
  line L673 (-80, 20) -> (-100, 20) construction
  line L674 (-61.5, 18.5) -> (-78.5, 18.5)
  line L675 (-61.5, 1.5) -> (-61.5, 18.5)
  line L676 (-78.5, 18.5) -> (-78.5, 1.5)
  line L677 (-78.5, 1.5) -> (-61.5, 1.5)
  line L678 (-60, 0) -> (-60, 20) construction
  line L679 (-60, 20) -> (-80, 20) construction
  line L680 (-41.5, 18.5) -> (-58.5, 18.5)
  line L681 (-41.5, 1.5) -> (-41.5, 18.5)
  line L682 (-58.5, 18.5) -> (-58.5, 1.5)
  line L683 (-58.5, 1.5) -> (-41.5, 1.5)
  line L684 (-40, 0) -> (-40, 20) construction
  line L685 (-40, 20) -> (-60, 20) construction
  line L686 (-21.5, 18.5) -> (-38.5, 18.5)
  line L687 (-21.5, 1.5) -> (-21.5, 18.5)
  line L688 (-38.5, 18.5) -> (-38.5, 1.5)
  line L689 (-38.5, 1.5) -> (-21.5, 1.5)
  line L690 (-20, 0) -> (-20, 20) construction
  line L691 (-20, 20) -> (-40, 20) construction
  line L692 (-1.5, 18.5) -> (-18.5, 18.5)
  line L693 (-1.5, 1.5) -> (-1.5, 18.5)
  line L694 (-18.5, 18.5) -> (-18.5, 1.5)
  line L695 (-18.5, 1.5) -> (-1.5, 1.5)
  line L696 (0, 0) -> (0, 20) construction
  line L697 (0, 20) -> (-20, 20) construction
  line L698 (18.5, 18.5) -> (1.5, 18.5)
  line L699 (18.5, 1.5) -> (18.5, 18.5)
  line L700 (1.5, 18.5) -> (1.5, 1.5)
  line L701 (1.5, 1.5) -> (18.5, 1.5)
  line L702 (20, 0) -> (20, 20) construction
  line L703 (20, 20) -> (0, 20) construction
  line L704 (38.5, 18.5) -> (21.5, 18.5)
  line L705 (38.5, 1.5) -> (38.5, 18.5)
  line L706 (21.5, 18.5) -> (21.5, 1.5)
  line L707 (21.5, 1.5) -> (38.5, 1.5)
  line L708 (40, 0) -> (40, 20) construction
  line L709 (40, 20) -> (20, 20) construction
  line L710 (58.5, 18.5) -> (41.5, 18.5)
  line L711 (58.5, 1.5) -> (58.5, 18.5)
  line L712 (41.5, 18.5) -> (41.5, 1.5)
  line L713 (41.5, 1.5) -> (58.5, 1.5)
  line L714 (60, 0) -> (60, 20) construction
  line L715 (60, 20) -> (40, 20) construction
  line L716 (78.5, 18.5) -> (61.5, 18.5)
  line L717 (78.5, 1.5) -> (78.5, 18.5)
  line L718 (61.5, 18.5) -> (61.5, 1.5)
  line L719 (61.5, 1.5) -> (78.5, 1.5)
  line L720 (80, 0) -> (80, 20) construction
  line L721 (80, 20) -> (60, 20) construction
  line L722 (98.5, 18.5) -> (81.5, 18.5)
  line L723 (98.5, 1.5) -> (98.5, 18.5)
  line L724 (81.5, 18.5) -> (81.5, 1.5)
  line L725 (81.5, 1.5) -> (98.5, 1.5)
  line L726 (100, 0) -> (100, 20) construction
  line L727 (100, 20) -> (80, 20) construction
  line L728 (-81.5, 38.5) -> (-98.5, 38.5)
  line L729 (-81.5, 21.5) -> (-81.5, 38.5)
  line L730 (-98.5, 38.5) -> (-98.5, 21.5)
  line L731 (-98.5, 21.5) -> (-81.5, 21.5)
  line L732 (-80, 20) -> (-80, 40) construction
  line L733 (-80, 40) -> (-100, 40) construction
  line L734 (-61.5, 38.5) -> (-78.5, 38.5)
  line L735 (-61.5, 21.5) -> (-61.5, 38.5)
  line L736 (-78.5, 38.5) -> (-78.5, 21.5)
  line L737 (-78.5, 21.5) -> (-61.5, 21.5)
  line L738 (-60, 20) -> (-60, 40) construction
  line L739 (-60, 40) -> (-80, 40) construction
  line L740 (-41.5, 38.5) -> (-58.5, 38.5)
  line L741 (-41.5, 21.5) -> (-41.5, 38.5)
  line L742 (-58.5, 38.5) -> (-58.5, 21.5)
  line L743 (-58.5, 21.5) -> (-41.5, 21.5)
  line L744 (-40, 20) -> (-40, 40) construction
  line L745 (-40, 40) -> (-60, 40) construction
  line L746 (-21.5, 38.5) -> (-38.5, 38.5)
  line L747 (-21.5, 21.5) -> (-21.5, 38.5)
  line L748 (-38.5, 38.5) -> (-38.5, 21.5)
  line L749 (-38.5, 21.5) -> (-21.5, 21.5)
  line L750 (-20, 20) -> (-20, 40) construction
  line L751 (-20, 40) -> (-40, 40) construction
  line L752 (-1.5, 38.5) -> (-18.5, 38.5)
  line L753 (-1.5, 21.5) -> (-1.5, 38.5)
  line L754 (-18.5, 38.5) -> (-18.5, 21.5)
  line L755 (-18.5, 21.5) -> (-1.5, 21.5)
  line L756 (0, 20) -> (0, 40) construction
  line L757 (0, 40) -> (-20, 40) construction
  line L758 (18.5, 38.5) -> (1.5, 38.5)
  line L759 (18.5, 21.5) -> (18.5, 38.5)
  line L760 (1.5, 38.5) -> (1.5, 21.5)
  line L761 (1.5, 21.5) -> (18.5, 21.5)
  line L762 (20, 20) -> (20, 40) construction
  line L763 (20, 40) -> (0, 40) construction
  line L764 (38.5, 38.5) -> (21.5, 38.5)
  line L765 (38.5, 21.5) -> (38.5, 38.5)
  line L766 (21.5, 38.5) -> (21.5, 21.5)
  line L767 (21.5, 21.5) -> (38.5, 21.5)
  line L768 (40, 20) -> (40, 40) construction
  line L769 (40, 40) -> (20, 40) construction
  line L770 (58.5, 38.5) -> (41.5, 38.5)
  line L771 (58.5, 21.5) -> (58.5, 38.5)
  line L772 (41.5, 38.5) -> (41.5, 21.5)
  line L773 (41.5, 21.5) -> (58.5, 21.5)
  line L774 (60, 20) -> (60, 40) construction
  line L775 (60, 40) -> (40, 40) construction
  line L776 (78.5, 38.5) -> (61.5, 38.5)
  line L777 (78.5, 21.5) -> (78.5, 38.5)
  line L778 (61.5, 38.5) -> (61.5, 21.5)
  line L779 (61.5, 21.5) -> (78.5, 21.5)
  line L780 (80, 20) -> (80, 40) construction
  line L781 (80, 40) -> (60, 40) construction
  line L782 (98.5, 38.5) -> (81.5, 38.5)
  line L783 (98.5, 21.5) -> (98.5, 38.5)
  line L784 (81.5, 38.5) -> (81.5, 21.5)
  line L785 (81.5, 21.5) -> (98.5, 21.5)
  line L786 (100, 20) -> (100, 40) construction
  line L787 (100, 40) -> (80, 40) construction
  line L788 (-81.5, 58.5) -> (-98.5, 58.5)
  line L789 (-81.5, 41.5) -> (-81.5, 58.5)
  line L790 (-98.5, 58.5) -> (-98.5, 41.5)
  line L791 (-98.5, 41.5) -> (-81.5, 41.5)
  line L792 (-80, 40) -> (-80, 60) construction
  line L793 (-80, 60) -> (-100, 60) construction
  line L794 (-61.5, 58.5) -> (-78.5, 58.5)
  line L795 (-61.5, 41.5) -> (-61.5, 58.5)
  line L796 (-78.5, 58.5) -> (-78.5, 41.5)
  line L797 (-78.5, 41.5) -> (-61.5, 41.5)
  line L798 (-60, 40) -> (-60, 60) construction
  line L799 (-60, 60) -> (-80, 60) construction
  line L800 (-41.5, 58.5) -> (-58.5, 58.5)
  line L801 (-41.5, 41.5) -> (-41.5, 58.5)
  line L802 (-58.5, 58.5) -> (-58.5, 41.5)
  line L803 (-58.5, 41.5) -> (-41.5, 41.5)
  line L804 (-40, 40) -> (-40, 60) construction
  line L805 (-40, 60) -> (-60, 60) construction
  line L806 (-21.5, 58.5) -> (-38.5, 58.5)
  line L807 (-21.5, 41.5) -> (-21.5, 58.5)
  line L808 (-38.5, 58.5) -> (-38.5, 41.5)
  line L809 (-38.5, 41.5) -> (-21.5, 41.5)
  line L810 (-20, 40) -> (-20, 60) construction
  line L811 (-20, 60) -> (-40, 60) construction
  line L812 (-1.5, 58.5) -> (-18.5, 58.5)
  line L813 (-1.5, 41.5) -> (-1.5, 58.5)
  line L814 (-18.5, 58.5) -> (-18.5, 41.5)
  line L815 (-18.5, 41.5) -> (-1.5, 41.5)
  line L816 (0, 40) -> (0, 60) construction
  line L817 (0, 60) -> (-20, 60) construction
  line L818 (18.5, 58.5) -> (1.5, 58.5)
  line L819 (18.5, 41.5) -> (18.5, 58.5)
  line L820 (1.5, 58.5) -> (1.5, 41.5)
  line L821 (1.5, 41.5) -> (18.5, 41.5)
  line L822 (20, 40) -> (20, 60) construction
  line L823 (20, 60) -> (0, 60) construction
  line L824 (38.5, 58.5) -> (21.5, 58.5)
  line L825 (38.5, 41.5) -> (38.5, 58.5)
  line L826 (21.5, 58.5) -> (21.5, 41.5)
  line L827 (21.5, 41.5) -> (38.5, 41.5)
  line L828 (40, 40) -> (40, 60) construction
  line L829 (40, 60) -> (20, 60) construction
  line L830 (58.5, 58.5) -> (41.5, 58.5)
  line L831 (58.5, 41.5) -> (58.5, 58.5)
  line L832 (41.5, 58.5) -> (41.5, 41.5)
  line L833 (41.5, 41.5) -> (58.5, 41.5)
  line L834 (60, 40) -> (60, 60) construction
  line L835 (60, 60) -> (40, 60) construction
  line L836 (78.5, 58.5) -> (61.5, 58.5)
  line L837 (78.5, 41.5) -> (78.5, 58.5)
  line L838 (61.5, 58.5) -> (61.5, 41.5)
  line L839 (61.5, 41.5) -> (78.5, 41.5)
  line L840 (80, 40) -> (80, 60) construction
  line L841 (80, 60) -> (60, 60) construction
  line L842 (98.5, 58.5) -> (81.5, 58.5)
  line L843 (98.5, 41.5) -> (98.5, 58.5)
  line L844 (81.5, 58.5) -> (81.5, 41.5)
  line L845 (81.5, 41.5) -> (98.5, 41.5)
  line L846 (100, 40) -> (100, 60) construction
  line L847 (100, 60) -> (80, 60) construction
  line L848 (-81.5, 78.5) -> (-98.5, 78.5)
  line L849 (-81.5, 61.5) -> (-81.5, 78.5)
  line L850 (-98.5, 78.5) -> (-98.5, 61.5)
  line L851 (-98.5, 61.5) -> (-81.5, 61.5)
  line L852 (-80, 60) -> (-80, 80) construction
  line L853 (-80, 80) -> (-100, 80) construction
  line L854 (-61.5, 78.5) -> (-78.5, 78.5)
  line L855 (-61.5, 61.5) -> (-61.5, 78.5)
  line L856 (-78.5, 78.5) -> (-78.5, 61.5)
  line L857 (-78.5, 61.5) -> (-61.5, 61.5)
  line L858 (-60, 60) -> (-60, 80) construction
  line L859 (-60, 80) -> (-80, 80) construction
  line L860 (-41.5, 78.5) -> (-58.5, 78.5)
  line L861 (-41.5, 61.5) -> (-41.5, 78.5)
  line L862 (-58.5, 78.5) -> (-58.5, 61.5)
  line L863 (-58.5, 61.5) -> (-41.5, 61.5)
  line L864 (-40, 60) -> (-40, 80) construction
  line L865 (-40, 80) -> (-60, 80) construction
  line L866 (-21.5, 78.5) -> (-38.5, 78.5)
  line L867 (-21.5, 61.5) -> (-21.5, 78.5)
  line L868 (-38.5, 78.5) -> (-38.5, 61.5)
  line L869 (-38.5, 61.5) -> (-21.5, 61.5)
  line L870 (-20, 60) -> (-20, 80) construction
  line L871 (-20, 80) -> (-40, 80) construction
  line L872 (-1.5, 78.5) -> (-18.5, 78.5)
  line L873 (-1.5, 61.5) -> (-1.5, 78.5)
  line L874 (-18.5, 78.5) -> (-18.5, 61.5)
  line L875 (-18.5, 61.5) -> (-1.5, 61.5)
  line L876 (0, 60) -> (0, 80) construction
  line L877 (0, 80) -> (-20, 80) construction
  line L878 (18.5, 78.5) -> (1.5, 78.5)
  line L879 (18.5, 61.5) -> (18.5, 78.5)
  line L880 (1.5, 78.5) -> (1.5, 61.5)
  line L881 (1.5, 61.5) -> (18.5, 61.5)
  line L882 (20, 60) -> (20, 80) construction
  line L883 (20, 80) -> (0, 80) construction
  line L884 (38.5, 78.5) -> (21.5, 78.5)
  line L885 (38.5, 61.5) -> (38.5, 78.5)
  line L886 (21.5, 78.5) -> (21.5, 61.5)
  line L887 (21.5, 61.5) -> (38.5, 61.5)
  line L888 (40, 60) -> (40, 80) construction
  line L889 (40, 80) -> (20, 80) construction
  line L890 (58.5, 78.5) -> (41.5, 78.5)
  line L891 (58.5, 61.5) -> (58.5, 78.5)
  line L892 (41.5, 78.5) -> (41.5, 61.5)
  line L893 (41.5, 61.5) -> (58.5, 61.5)
  line L894 (60, 60) -> (60, 80) construction
  line L895 (60, 80) -> (40, 80) construction
  line L896 (78.5, 78.5) -> (61.5, 78.5)
  line L897 (78.5, 61.5) -> (78.5, 78.5)
  line L898 (61.5, 78.5) -> (61.5, 61.5)
  line L899 (61.5, 61.5) -> (78.5, 61.5)
  line L900 (80, 60) -> (80, 80) construction
  line L901 (80, 80) -> (60, 80) construction
  line L902 (98.5, 78.5) -> (81.5, 78.5)
  line L903 (98.5, 61.5) -> (98.5, 78.5)
  line L904 (81.5, 78.5) -> (81.5, 61.5)
  line L905 (81.5, 61.5) -> (98.5, 61.5)
  line L906 (100, 60) -> (100, 80) construction
  line L907 (100, 80) -> (80, 80) construction
  line L908 (-81.5, 98.5) -> (-98.5, 98.5)
  line L909 (-81.5, 81.5) -> (-81.5, 98.5)
  line L910 (-98.5, 98.5) -> (-98.5, 81.5)
  line L911 (-98.5, 81.5) -> (-81.5, 81.5)
  line L912 (-80, 80) -> (-80, 100) construction
  line L913 (-80, 100) -> (-100, 100) construction
  line L914 (-61.5, 98.5) -> (-78.5, 98.5)
  line L915 (-61.5, 81.5) -> (-61.5, 98.5)
  line L916 (-78.5, 98.5) -> (-78.5, 81.5)
  line L917 (-78.5, 81.5) -> (-61.5, 81.5)
  line L918 (-60, 80) -> (-60, 100) construction
  line L919 (-60, 100) -> (-80, 100) construction
  line L920 (-41.5, 98.5) -> (-58.5, 98.5)
  line L921 (-41.5, 81.5) -> (-41.5, 98.5)
  line L922 (-58.5, 98.5) -> (-58.5, 81.5)
  line L923 (-58.5, 81.5) -> (-41.5, 81.5)
  line L924 (-40, 80) -> (-40, 100) construction
  line L925 (-40, 100) -> (-60, 100) construction
  line L926 (-21.5, 98.5) -> (-38.5, 98.5)
  line L927 (-21.5, 81.5) -> (-21.5, 98.5)
  line L928 (-38.5, 98.5) -> (-38.5, 81.5)
  line L929 (-38.5, 81.5) -> (-21.5, 81.5)
  line L930 (-20, 80) -> (-20, 100) construction
  line L931 (-20, 100) -> (-40, 100) construction
  line L932 (-1.5, 98.5) -> (-18.5, 98.5)
  line L933 (-1.5, 81.5) -> (-1.5, 98.5)
  line L934 (-18.5, 98.5) -> (-18.5, 81.5)
  line L935 (-18.5, 81.5) -> (-1.5, 81.5)
  line L936 (0, 80) -> (0, 100) construction
  line L937 (0, 100) -> (-20, 100) construction
  line L938 (18.5, 98.5) -> (1.5, 98.5)
  line L939 (18.5, 81.5) -> (18.5, 98.5)
  line L940 (1.5, 98.5) -> (1.5, 81.5)
  line L941 (1.5, 81.5) -> (18.5, 81.5)
  line L942 (20, 80) -> (20, 100) construction
  line L943 (20, 100) -> (0, 100) construction
  line L944 (38.5, 98.5) -> (21.5, 98.5)
  line L945 (38.5, 81.5) -> (38.5, 98.5)
  line L946 (21.5, 98.5) -> (21.5, 81.5)
  line L947 (21.5, 81.5) -> (38.5, 81.5)
  line L948 (40, 80) -> (40, 100) construction
  line L949 (40, 100) -> (20, 100) construction
  line L950 (58.5, 98.5) -> (41.5, 98.5)
  line L951 (58.5, 81.5) -> (58.5, 98.5)
  line L952 (41.5, 98.5) -> (41.5, 81.5)
  line L953 (41.5, 81.5) -> (58.5, 81.5)
  line L954 (60, 80) -> (60, 100) construction
  line L955 (60, 100) -> (40, 100) construction
  line L956 (78.5, 98.5) -> (61.5, 98.5)
  line L957 (78.5, 81.5) -> (78.5, 98.5)
  line L958 (61.5, 98.5) -> (61.5, 81.5)
  line L959 (61.5, 81.5) -> (78.5, 81.5)
  line L960 (80, 80) -> (80, 100) construction
  line L961 (80, 100) -> (60, 100) construction
  line L962 (98.5, 98.5) -> (81.5, 98.5)
  line L963 (98.5, 81.5) -> (98.5, 98.5)
  line L964 (81.5, 98.5) -> (81.5, 81.5)
  line L965 (81.5, 81.5) -> (98.5, 81.5)
  line L966 (100, 80) -> (100, 100) construction
  line L967 (100, 100) -> (80, 100) construction
  line L968 (-81.5, 118.5) -> (-98.5, 118.5)
  line L969 (-81.5, 101.5) -> (-81.5, 118.5)
  line L970 (-98.5, 118.5) -> (-98.5, 101.5)
  line L971 (-98.5, 101.5) -> (-81.5, 101.5)
  line L972 (-80, 100) -> (-80, 120) construction
  line L973 (-80, 120) -> (-100, 120) construction
  line L974 (-61.5, 118.5) -> (-78.5, 118.5)
  line L975 (-61.5, 101.5) -> (-61.5, 118.5)
  line L976 (-78.5, 118.5) -> (-78.5, 101.5)
  line L977 (-78.5, 101.5) -> (-61.5, 101.5)
  line L978 (-60, 100) -> (-60, 120) construction
  line L979 (-60, 120) -> (-80, 120) construction
  line L980 (-41.5, 118.5) -> (-58.5, 118.5)
  line L981 (-41.5, 101.5) -> (-41.5, 118.5)
  line L982 (-58.5, 118.5) -> (-58.5, 101.5)
  line L983 (-58.5, 101.5) -> (-41.5, 101.5)
  line L984 (-40, 100) -> (-40, 120) construction
  line L985 (-40, 120) -> (-60, 120) construction
  line L986 (-21.5, 118.5) -> (-38.5, 118.5)
  line L987 (-21.5, 101.5) -> (-21.5, 118.5)
  line L988 (-38.5, 118.5) -> (-38.5, 101.5)
  line L989 (-38.5, 101.5) -> (-21.5, 101.5)
  line L990 (-20, 100) -> (-20, 120) construction
  line L991 (-20, 120) -> (-40, 120) construction
  line L992 (-1.5, 118.5) -> (-18.5, 118.5)
  line L993 (-1.5, 101.5) -> (-1.5, 118.5)
  line L994 (-18.5, 118.5) -> (-18.5, 101.5)
  line L995 (-18.5, 101.5) -> (-1.5, 101.5)
  line L996 (0, 100) -> (0, 120) construction
  line L997 (0, 120) -> (-20, 120) construction
  line L998 (18.5, 118.5) -> (1.5, 118.5)
  line L999 (18.5, 101.5) -> (18.5, 118.5)
  line L1000 (1.5, 118.5) -> (1.5, 101.5)
  line L1001 (1.5, 101.5) -> (18.5, 101.5)
  line L1002 (20, 100) -> (20, 120) construction
  line L1003 (20, 120) -> (0, 120) construction
  line L1004 (38.5, 118.5) -> (21.5, 118.5)
  line L1005 (38.5, 101.5) -> (38.5, 118.5)
  line L1006 (21.5, 118.5) -> (21.5, 101.5)
  line L1007 (21.5, 101.5) -> (38.5, 101.5)
  line L1008 (40, 100) -> (40, 120) construction
  line L1009 (40, 120) -> (20, 120) construction
  line L1010 (58.5, 118.5) -> (41.5, 118.5)
  line L1011 (58.5, 101.5) -> (58.5, 118.5)
  line L1012 (41.5, 118.5) -> (41.5, 101.5)
  line L1013 (41.5, 101.5) -> (58.5, 101.5)
  line L1014 (60, 100) -> (60, 120) construction
  line L1015 (60, 120) -> (40, 120) construction
  line L1016 (78.5, 118.5) -> (61.5, 118.5)
  line L1017 (78.5, 101.5) -> (78.5, 118.5)
  line L1018 (61.5, 118.5) -> (61.5, 101.5)
  line L1019 (61.5, 101.5) -> (78.5, 101.5)
  line L1020 (80, 100) -> (80, 120) construction
  line L1021 (80, 120) -> (60, 120) construction
  line L1022 (98.5, 118.5) -> (81.5, 118.5)
  line L1023 (98.5, 101.5) -> (98.5, 118.5)
  line L1024 (81.5, 118.5) -> (81.5, 101.5)
  line L1025 (81.5, 101.5) -> (98.5, 101.5)
  line L1026 (100, 100) -> (100, 120) construction
  line L1027 (100, 120) -> (80, 120) construction
  line L1028 (-81.5, 138.5) -> (-98.5, 138.5)
  line L1029 (-81.5, 121.5) -> (-81.5, 138.5)
  line L1030 (-98.5, 138.5) -> (-98.5, 121.5)
  line L1031 (-98.5, 121.5) -> (-81.5, 121.5)
  line L1032 (-80, 120) -> (-80, 140) construction
  line L1033 (-80, 140) -> (-100, 140) construction
  line L1034 (-61.5, 138.5) -> (-78.5, 138.5)
  line L1035 (-61.5, 121.5) -> (-61.5, 138.5)
  line L1036 (-78.5, 138.5) -> (-78.5, 121.5)
  line L1037 (-78.5, 121.5) -> (-61.5, 121.5)
  line L1038 (-60, 120) -> (-60, 140) construction
  line L1039 (-60, 140) -> (-80, 140) construction
  line L1040 (-41.5, 138.5) -> (-58.5, 138.5)
  line L1041 (-41.5, 121.5) -> (-41.5, 138.5)
  line L1042 (-58.5, 138.5) -> (-58.5, 121.5)
  line L1043 (-58.5, 121.5) -> (-41.5, 121.5)
  line L1044 (-40, 120) -> (-40, 140) construction
  line L1045 (-40, 140) -> (-60, 140) construction
  line L1046 (-21.5, 138.5) -> (-38.5, 138.5)
  line L1047 (-21.5, 121.5) -> (-21.5, 138.5)
  line L1048 (-38.5, 138.5) -> (-38.5, 121.5)
  line L1049 (-38.5, 121.5) -> (-21.5, 121.5)
  line L1050 (-20, 120) -> (-20, 140) construction
  line L1051 (-20, 140) -> (-40, 140) construction
  line L1052 (-1.5, 138.5) -> (-18.5, 138.5)
  line L1053 (-1.5, 121.5) -> (-1.5, 138.5)
  line L1054 (-18.5, 138.5) -> (-18.5, 121.5)
  line L1055 (-18.5, 121.5) -> (-1.5, 121.5)
  line L1056 (0, 120) -> (0, 140) construction
  line L1057 (0, 140) -> (-20, 140) construction
  line L1058 (18.5, 138.5) -> (1.5, 138.5)
  line L1059 (18.5, 121.5) -> (18.5, 138.5)
  line L1060 (1.5, 138.5) -> (1.5, 121.5)
  line L1061 (1.5, 121.5) -> (18.5, 121.5)
  line L1062 (20, 120) -> (20, 140) construction
  line L1063 (20, 140) -> (0, 140) construction
  line L1064 (38.5, 138.5) -> (21.5, 138.5)
  line L1065 (38.5, 121.5) -> (38.5, 138.5)
  line L1066 (21.5, 138.5) -> (21.5, 121.5)
  line L1067 (21.5, 121.5) -> (38.5, 121.5)
  line L1068 (40, 120) -> (40, 140) construction
  line L1069 (40, 140) -> (20, 140) construction
  line L1070 (58.5, 138.5) -> (41.5, 138.5)
  line L1071 (58.5, 121.5) -> (58.5, 138.5)
  line L1072 (41.5, 138.5) -> (41.5, 121.5)
  line L1073 (41.5, 121.5) -> (58.5, 121.5)
  line L1074 (60, 120) -> (60, 140) construction
  line L1075 (60, 140) -> (40, 140) construction
  line L1076 (78.5, 138.5) -> (61.5, 138.5)
  line L1077 (78.5, 121.5) -> (78.5, 138.5)
  line L1078 (61.5, 138.5) -> (61.5, 121.5)
  line L1079 (61.5, 121.5) -> (78.5, 121.5)
  line L1080 (80, 120) -> (80, 140) construction
  line L1081 (80, 140) -> (60, 140) construction
  line L1082 (98.5, 138.5) -> (81.5, 138.5)
  line L1083 (98.5, 121.5) -> (98.5, 138.5)
  line L1084 (81.5, 138.5) -> (81.5, 121.5)
  line L1085 (81.5, 121.5) -> (98.5, 121.5)
  line L1086 (100, 120) -> (100, 140) construction
  line L1087 (100, 140) -> (80, 140) construction
  line L1088 (-81.5, 158.5) -> (-98.5, 158.5)
  line L1089 (-81.5, 141.5) -> (-81.5, 158.5)
  line L1090 (-98.5, 158.5) -> (-98.5, 141.5)
  line L1091 (-98.5, 141.5) -> (-81.5, 141.5)
  line L1092 (-80, 140) -> (-80, 160) construction